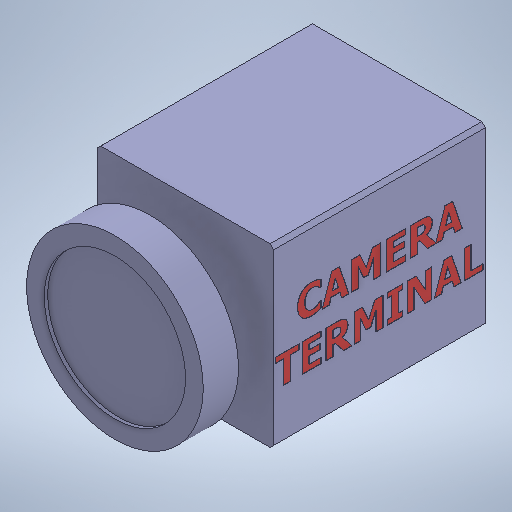
# Autodesk Inventor part: CAMERA
Saved by Autodesk Inventor 2025 (Build 290162000, 162)
## iProperties
Created: 2024-09-26
Part Number: CAMERA
Material: ABS Plastic
Document SubType Name: Modeling
Designer: DMIADX
Density: 1.06 g/cm^3
Appearance: Slate Blue
Author: DMIADX
Autodesk Inventor part; units mm, degrees
ref_plane "YZ Plane" through (0, 0, 0) normal (1, 0, 0) x (0, 1, 0)
ref_plane "XZ Plane" through (0, 0, 0) normal (0, 1, 0) x (-1, 0, 0)
ref_plane "XY Plane" through (0, 0, 0) normal (0, 0, 1) x (1, 0, 0)
sketch "Sketch1" plane through (0, 0, 0) normal (0, 0, 1) x (1, 0, 0)
  line L0 (25, -25) -> (-25, -25)
  line L1 (-25, -25) -> (-25, 25)
  line L2 (-25, 25) -> (25, 25)
  line L3 (25, 25) -> (25, -25)
  line L4 (25, -25) -> (-25, 25) construction
  line L5 (-25, -25) -> (25, 25) construction
  point P0 (0, 0)
  dimension "d0" = 50
  dimension "d1" = 50
  constraints: 12 end point, 2 midpoint, 2 parallel, 1 horizontal, 1 perpendicular
  measures "d0" distance of L0.end L1.end
  measures "d1" distance of L1.end L2.end
extrude "Extrusion1" add sketch "Sketch1" along normal blind 60
chamfer "Chamfer1" distance 1 angle 45 4 edges at (25, 25, 30) (-25, 25, 30) (-25, -25, 30) (25, -25, 30)
sketch "Sketch2" plane through (0, 0, 60) normal (0, 0, 1) x (1, 0, 0)
  circle A0 centre (0, 0) radius 25
  line L0 (24, 25) -> (-24, 25) projected
  circle A1 centre (0, 0) radius 10
  dimension "d7" = 20
  constraints: 2 centre point, 2 coincident, 1 tangent
  measures "d7" diameter of A1
extrude "Extrusion2" add sketch "Sketch2" along normal blind 20 contours A0 | A1
extrude "Extrusion3" cut sketch "Sketch2" along normal blind 10
sketch "Sketch3" plane through (0, 0, 80) normal (0, 0, 1) x (1, 0, 0)
  circle A0 centre (0, 0) radius 20
  constraints: 1 centre point, 1 coincident
extrude "Extrusion4" cut sketch "Sketch3" against normal blind 1
sketch "Sketch4" plane through (25, -24, 0) normal (1, 0, 0) x (0, 0, -1)
  line L0 (-60, 49) -> (0, 49) construction
  line L1 (0, 49) -> (0, -1) construction
  line L2 (0, -1) -> (-60, -1) construction
  line L3 (-60, -1) -> (-60, 49) construction
  line L4 (0, 0) -> (0, 48) projected
  spline S0 degree 2 poles (-49.2512, 26.3525) (-51.0535, 26.3525) (-53.1669, 28.5308) (-53.1669, 30.5016) knots 0 0 0 1 2 2 2
  spline S1 degree 2 poles (-53.1669, 30.5016) (-53.1669, 32.4011) (-51.047, 34.6637) (-49.2447, 34.6637) knots 0 0 0 1 2 2 2
  spline S2 degree 2 poles (-49.2447, 34.6637) (-48.7715, 34.6637) (-48.0065, 34.5535) (-47.6564, 34.4627) knots 0 0 0 1 2 2 2
  spline S3 degree 2 poles (-47.6564, 34.4627) (-47.3841, 34.3784) (-46.7423, 34.0997) (-46.5413, 33.9959) knots 0 0 0 1 2 2 2
  line L5 (-46.5413, 33.9959) -> (-46.5413, 32.0899)
  line L6 (-46.5413, 32.0899) -> (-46.7423, 32.0899)
  spline S4 degree 2 poles (-46.7423, 32.0899) (-46.8914, 32.2196) (-47.3323, 32.5827) (-47.611, 32.7512) knots 0 0 0 1 2 2 2
  spline S5 degree 2 poles (-47.611, 32.7512) (-47.8898, 32.9263) (-48.5575, 33.1661) (-48.9271, 33.1661) knots 0 0 0 1 2 2 2
  spline S6 degree 2 poles (-48.9271, 33.1661) (-49.3614, 33.1661) (-50.081, 32.8938) (-50.4117, 32.5502) knots 0 0 0 1 2 2 2
  spline S7 degree 2 poles (-50.4117, 32.5502) (-50.7099, 32.2455) (-51.0924, 31.2018) (-51.0924, 30.4951) knots 0 0 0 1 2 2 2
  spline S8 degree 2 poles (-51.0924, 30.4951) (-51.0924, 29.7496) (-50.6969, 28.7318) (-50.3728, 28.4206) knots 0 0 0 1 2 2 2
  spline S9 degree 2 poles (-50.3728, 28.4206) (-50.0616, 28.1159) (-49.2966, 27.8501) (-48.9141, 27.8501) knots 0 0 0 1 2 2 2
  spline S10 degree 2 poles (-48.9141, 27.8501) (-48.5186, 27.8501) (-47.799, 28.1159) (-47.5527, 28.278) knots 0 0 0 1 2 2 2
  spline S11 degree 2 poles (-47.5527, 28.278) (-47.2804, 28.44) (-46.872, 28.7836) (-46.7229, 28.9198) knots 0 0 0 1 2 2 2
  line L7 (-46.7229, 28.9198) -> (-46.5413, 28.9198)
  line L8 (-46.5413, 28.9198) -> (-46.5413, 27.0397)
  spline S12 degree 2 poles (-46.5413, 27.0397) (-46.7618, 26.936) (-47.3387, 26.6767) (-47.6499, 26.5859) knots 0 0 0 1 2 2 2
  spline S13 degree 2 poles (-47.6499, 26.5859) (-48.0259, 26.4692) (-48.6807, 26.3525) (-49.2512, 26.3525) knots 0 0 0 1 2 2 2
  line L9 (-46.2172, 26.5081) -> (-43.5138, 34.5081)
  line L10 (-43.5138, 34.5081) -> (-41.3225, 34.5081)
  line L11 (-41.3225, 34.5081) -> (-38.6191, 26.5081)
  line L12 (-38.6191, 26.5081) -> (-40.6872, 26.5081)
  line L13 (-40.6872, 26.5081) -> (-41.1864, 28.1418)
  line L14 (-41.1864, 28.1418) -> (-43.7018, 28.1418)
  line L15 (-43.7018, 28.1418) -> (-44.2075, 26.5081)
  line L16 (-44.2075, 26.5081) -> (-46.2172, 26.5081)
  line L17 (-41.6272, 29.594) -> (-42.4441, 32.2391)
  line L18 (-42.4441, 32.2391) -> (-43.2674, 29.594)
  line L19 (-43.2674, 29.594) -> (-41.6272, 29.594)
  line L20 (-29.6532, 26.5081) -> (-31.6499, 26.5081)
  line L21 (-31.6499, 26.5081) -> (-31.6499, 31.8112)
  line L22 (-31.6499, 31.8112) -> (-33.1021, 28.3882)
  line L23 (-33.1021, 28.3882) -> (-34.4765, 28.3882)
  line L24 (-34.4765, 28.3882) -> (-35.9287, 31.8112)
  line L25 (-35.9287, 31.8112) -> (-35.9287, 26.5081)
  line L26 (-35.9287, 26.5081) -> (-37.8217, 26.5081)
  line L27 (-37.8217, 26.5081) -> (-37.8217, 34.5081)
  line L28 (-37.8217, 34.5081) -> (-35.5073, 34.5081)
  line L29 (-35.5073, 34.5081) -> (-33.731, 30.56)
  line L30 (-33.731, 30.56) -> (-31.9676, 34.5081)
  line L31 (-31.9676, 34.5081) -> (-29.6532, 34.5081)
  line L32 (-29.6532, 34.5081) -> (-29.6532, 26.5081)
  line L33 (-27.9935, 26.5081) -> (-27.9935, 34.5081)
  line L34 (-27.9935, 34.5081) -> (-22.5867, 34.5081)
  line L35 (-22.5867, 34.5081) -> (-22.5867, 32.9846)
  line L36 (-22.5867, 32.9846) -> (-25.9968, 32.9846)
  line L37 (-25.9968, 32.9846) -> (-25.9968, 31.5778)
  line L38 (-25.9968, 31.5778) -> (-22.8525, 31.5778)
  line L39 (-22.8525, 31.5778) -> (-22.8525, 30.0543)
  line L40 (-22.8525, 30.0543) -> (-25.9968, 30.0543)
  line L41 (-25.9968, 30.0543) -> (-25.9968, 28.0316)
  line L42 (-25.9968, 28.0316) -> (-22.5867, 28.0316)
  line L43 (-22.5867, 28.0316) -> (-22.5867, 26.5081)
  line L44 (-22.5867, 26.5081) -> (-27.9935, 26.5081)
  line L45 (-13.8347, 26.5081) -> (-16.2788, 26.5081)
  line L46 (-16.2788, 26.5081) -> (-18.5024, 29.4449)
  line L47 (-18.5024, 29.4449) -> (-19.2285, 29.4449)
  line L48 (-19.2285, 29.4449) -> (-19.2285, 26.5081)
  line L49 (-19.2285, 26.5081) -> (-21.2253, 26.5081)
  line L50 (-21.2253, 26.5081) -> (-21.2253, 34.5081)
  line L51 (-21.2253, 34.5081) -> (-18.0097, 34.5081)
  spline S14 degree 2 poles (-18.0097, 34.5081) (-17.342, 34.5081) (-16.3566, 34.3395) (-15.9352, 34.0802) knots 0 0 0 1 2 2 2
  spline S15 degree 2 poles (-15.9352, 34.0802) (-15.5073, 33.8079) (-15.0016, 32.9587) (-15.0016, 32.3104) knots 0 0 0 1 2 2 2
  spline S16 degree 2 poles (-15.0016, 32.3104) (-15.0016, 31.3963) (-15.8314, 30.2488) (-16.5251, 29.9117) knots 0 0 0 1 2 2 2
  line L52 (-16.5251, 29.9117) -> (-13.8347, 26.5081)
  spline S17 degree 2 poles (-17.0632, 32.0575) (-17.0632, 32.3622) (-17.2966, 32.7966) (-17.5624, 32.9133) knots 0 0 0 1 2 2 2
  spline S18 degree 2 poles (-17.5624, 32.9133) (-17.7504, 32.9911) (-18.2107, 33.0365) (-18.5543, 33.0365) knots 0 0 0 1 2 2 2
  line L53 (-18.5543, 33.0365) -> (-19.2285, 33.0365)
  line L54 (-19.2285, 33.0365) -> (-19.2285, 30.8841)
  line L55 (-19.2285, 30.8841) -> (-18.6515, 30.8841)
  spline S19 degree 2 poles (-18.6515, 30.8841) (-18.2366, 30.8841) (-17.6467, 30.9878) (-17.4457, 31.1499) knots 0 0 0 1 2 2 2
  spline S20 degree 2 poles (-17.4457, 31.1499) (-17.2512, 31.3055) (-17.0632, 31.7204) (-17.0632, 32.0575) knots 0 0 0 1 2 2 2
  line L56 (-14.1005, 26.5081) -> (-11.3971, 34.5081)
  line L57 (-11.3971, 34.5081) -> (-9.2058, 34.5081)
  line L58 (-9.2058, 34.5081) -> (-6.5024, 26.5081)
  line L59 (-6.5024, 26.5081) -> (-8.5705, 26.5081)
  line L60 (-8.5705, 26.5081) -> (-9.0697, 28.1418)
  line L61 (-9.0697, 28.1418) -> (-11.5851, 28.1418)
  line L62 (-11.5851, 28.1418) -> (-12.0908, 26.5081)
  line L63 (-12.0908, 26.5081) -> (-14.1005, 26.5081)
  line L64 (-9.5105, 29.594) -> (-10.3274, 32.2391)
  line L65 (-10.3274, 32.2391) -> (-11.1507, 29.594)
  line L66 (-11.1507, 29.594) -> (-9.5105, 29.594)
  line L67 (-57.1053, 13.3363) -> (-57.1053, 19.8128)
  line L68 (-57.1053, 19.8128) -> (-59.4716, 19.8128)
  line L69 (-59.4716, 19.8128) -> (-59.4716, 21.3363)
  line L70 (-59.4716, 21.3363) -> (-52.7293, 21.3363)
  line L71 (-52.7293, 21.3363) -> (-52.7293, 19.8128)
  line L72 (-52.7293, 19.8128) -> (-55.0956, 19.8128)
  line L73 (-55.0956, 19.8128) -> (-55.0956, 13.3363)
  line L74 (-55.0956, 13.3363) -> (-57.1053, 13.3363)
  line L75 (-51.906, 13.3363) -> (-51.906, 21.3363)
  line L76 (-51.906, 21.3363) -> (-46.4992, 21.3363)
  line L77 (-46.4992, 21.3363) -> (-46.4992, 19.8128)
  line L78 (-46.4992, 19.8128) -> (-49.9092, 19.8128)
  line L79 (-49.9092, 19.8128) -> (-49.9092, 18.406)
  line L80 (-49.9092, 18.406) -> (-46.765, 18.406)
  line L81 (-46.765, 18.406) -> (-46.765, 16.8825)
  line L82 (-46.765, 16.8825) -> (-49.9092, 16.8825)
  line L83 (-49.9092, 16.8825) -> (-49.9092, 14.8598)
  line L84 (-49.9092, 14.8598) -> (-46.4992, 14.8598)
  line L85 (-46.4992, 14.8598) -> (-46.4992, 13.3363)
  line L86 (-46.4992, 13.3363) -> (-51.906, 13.3363)
  line L87 (-37.7472, 13.3363) -> (-40.1912, 13.3363)
  line L88 (-40.1912, 13.3363) -> (-42.4149, 16.2731)
  line L89 (-42.4149, 16.2731) -> (-43.141, 16.2731)
  line L90 (-43.141, 16.2731) -> (-43.141, 13.3363)
  line L91 (-43.141, 13.3363) -> (-45.1378, 13.3363)
  line L92 (-45.1378, 13.3363) -> (-45.1378, 21.3363)
  line L93 (-45.1378, 21.3363) -> (-41.9222, 21.3363)
  spline S21 degree 2 poles (-41.9222, 21.3363) (-41.2545, 21.3363) (-40.269, 21.1678) (-39.8477, 20.9084) knots 0 0 0 1 2 2 2
  spline S22 degree 2 poles (-39.8477, 20.9084) (-39.4198, 20.6361) (-38.9141, 19.7869) (-38.9141, 19.1386) knots 0 0 0 1 2 2 2
  spline S23 degree 2 poles (-38.9141, 19.1386) (-38.9141, 18.2245) (-39.7439, 17.077) (-40.4376, 16.7399) knots 0 0 0 1 2 2 2
  line L94 (-40.4376, 16.7399) -> (-37.7472, 13.3363)
  spline S24 degree 2 poles (-40.9757, 18.8857) (-40.9757, 19.1904) (-41.2091, 19.6248) (-41.4749, 19.7415) knots 0 0 0 1 2 2 2
  spline S25 degree 2 poles (-41.4749, 19.7415) (-41.6629, 19.8193) (-42.1232, 19.8647) (-42.4668, 19.8647) knots 0 0 0 1 2 2 2
  line L95 (-42.4668, 19.8647) -> (-43.141, 19.8647)
  line L96 (-43.141, 19.8647) -> (-43.141, 17.7123)
  line L97 (-43.141, 17.7123) -> (-42.564, 17.7123)
  spline S26 degree 2 poles (-42.564, 17.7123) (-42.1491, 17.7123) (-41.5592, 17.8161) (-41.3582, 17.9781) knots 0 0 0 1 2 2 2
  spline S27 degree 2 poles (-41.3582, 17.9781) (-41.1637, 18.1337) (-40.9757, 18.5486) (-40.9757, 18.8857) knots 0 0 0 1 2 2 2
  line L98 (-28.9822, 13.3363) -> (-30.9789, 13.3363)
  line L99 (-30.9789, 13.3363) -> (-30.9789, 18.6394)
  line L100 (-30.9789, 18.6394) -> (-32.4311, 15.2164)
  line L101 (-32.4311, 15.2164) -> (-33.8055, 15.2164)
  line L102 (-33.8055, 15.2164) -> (-35.2577, 18.6394)
  line L103 (-35.2577, 18.6394) -> (-35.2577, 13.3363)
  line L104 (-35.2577, 13.3363) -> (-37.1507, 13.3363)
  line L105 (-37.1507, 13.3363) -> (-37.1507, 21.3363)
  line L106 (-37.1507, 21.3363) -> (-34.8363, 21.3363)
  line L107 (-34.8363, 21.3363) -> (-33.06, 17.3882)
  line L108 (-33.06, 17.3882) -> (-31.2966, 21.3363)
  line L109 (-31.2966, 21.3363) -> (-28.9822, 21.3363)
  line L110 (-28.9822, 21.3363) -> (-28.9822, 13.3363)
  line L111 (-23.342, 13.3363) -> (-27.6467, 13.3363)
  line L112 (-27.6467, 13.3363) -> (-27.6467, 14.7302)
  line L113 (-27.6467, 14.7302) -> (-26.4992, 14.7302)
  line L114 (-26.4992, 14.7302) -> (-26.4992, 19.9425)
  line L115 (-26.4992, 19.9425) -> (-27.6467, 19.9425)
  line L116 (-27.6467, 19.9425) -> (-27.6467, 21.3363)
  line L117 (-27.6467, 21.3363) -> (-23.342, 21.3363)
  line L118 (-23.342, 21.3363) -> (-23.342, 19.9425)
  line L119 (-23.342, 19.9425) -> (-24.4895, 19.9425)
  line L120 (-24.4895, 19.9425) -> (-24.4895, 14.7302)
  line L121 (-24.4895, 14.7302) -> (-23.342, 14.7302)
  line L122 (-23.342, 14.7302) -> (-23.342, 13.3363)
  line L123 (-15.154, 13.3363) -> (-17.0859, 13.3363)
  line L124 (-17.0859, 13.3363) -> (-20.1718, 18.9117)
  line L125 (-20.1718, 18.9117) -> (-20.1718, 13.3363)
  line L126 (-20.1718, 13.3363) -> (-22.0065, 13.3363)
  line L127 (-22.0065, 13.3363) -> (-22.0065, 21.3363)
  line L128 (-22.0065, 21.3363) -> (-19.543, 21.3363)
  line L129 (-19.543, 21.3363) -> (-16.9887, 16.7528)
  line L130 (-16.9887, 16.7528) -> (-16.9887, 21.3363)
  line L131 (-16.9887, 21.3363) -> (-15.154, 21.3363)
  line L132 (-15.154, 21.3363) -> (-15.154, 13.3363)
  line L133 (-14.389, 13.3363) -> (-11.6856, 21.3363)
  line L134 (-11.6856, 21.3363) -> (-9.4943, 21.3363)
  line L135 (-9.4943, 21.3363) -> (-6.7909, 13.3363)
  line L136 (-6.7909, 13.3363) -> (-8.859, 13.3363)
  line L137 (-8.859, 13.3363) -> (-9.3582, 14.97)
  line L138 (-9.3582, 14.97) -> (-11.8736, 14.97)
  line L139 (-11.8736, 14.97) -> (-12.3793, 13.3363)
  line L140 (-12.3793, 13.3363) -> (-14.389, 13.3363)
  line L141 (-9.799, 16.4222) -> (-10.6159, 19.0673)
  line L142 (-10.6159, 19.0673) -> (-11.4392, 16.4222)
  line L143 (-11.4392, 16.4222) -> (-9.799, 16.4222)
  line L144 (-0.658, 13.3363) -> (-5.9935, 13.3363)
  line L145 (-5.9935, 13.3363) -> (-5.9935, 21.3363)
  line L146 (-5.9935, 21.3363) -> (-3.9838, 21.3363)
  line L147 (-3.9838, 21.3363) -> (-3.9838, 14.8598)
  line L148 (-3.9838, 14.8598) -> (-0.658, 14.8598)
  line L149 (-0.658, 14.8598) -> (-0.658, 13.3363)
  point P0 (0, 24)
  point P1 (0, 24)
  point P2 (0, 24)
  dimension "d14" = 60
  dimension "d15" = 0
  dimension "d16" = 50
  dimension "d17" = 25
  constraints: 2 midpoint, 2 other
  measures "d14" distance of L1.end L2.end
  measures "d15" horizontal distance of point (0, 24) L1.end
  measures "d16" distance between parallel lines of L2 L0
  measures "d17" distance from line of point (0, 24) L0
emboss "Emboss1" sketch "Sketch4" operation cut depth 0.1 direction (-1, 0, 0)
sketch "Sketch5" plane through (-25, -24, 0) normal (-1, 0, 0) x (0, 0, 1)
  line L0 (0, 49) -> (60, 49) construction
  line L1 (60, 49) -> (60, -1) construction
  line L2 (60, -1) -> (0, -1) construction
  line L3 (0, -1) -> (0, 49) construction
  line L4 (0, -1) -> (60, -1) projected
  line L5 (60, 48) -> (60, 0) projected
  spline S0 degree 2 poles (10.7488, 26.3525) (8.9465, 26.3525) (6.8331, 28.5308) (6.8331, 30.5016) knots 0 0 0 1 2 2 2
  spline S1 degree 2 poles (6.8331, 30.5016) (6.8331, 32.4011) (8.953, 34.6637) (10.7553, 34.6637) knots 0 0 0 1 2 2 2
  spline S2 degree 2 poles (10.7553, 34.6637) (11.2285, 34.6637) (11.9935, 34.5535) (12.3436, 34.4627) knots 0 0 0 1 2 2 2
  spline S3 degree 2 poles (12.3436, 34.4627) (12.6159, 34.3784) (13.2577, 34.0997) (13.4587, 33.9959) knots 0 0 0 1 2 2 2
  line L6 (13.4587, 33.9959) -> (13.4587, 32.0899)
  line L7 (13.4587, 32.0899) -> (13.2577, 32.0899)
  spline S4 degree 2 poles (13.2577, 32.0899) (13.1086, 32.2196) (12.6677, 32.5827) (12.389, 32.7512) knots 0 0 0 1 2 2 2
  spline S5 degree 2 poles (12.389, 32.7512) (12.1102, 32.9263) (11.4425, 33.1661) (11.0729, 33.1661) knots 0 0 0 1 2 2 2
  spline S6 degree 2 poles (11.0729, 33.1661) (10.6386, 33.1661) (9.919, 32.8938) (9.5883, 32.5502) knots 0 0 0 1 2 2 2
  spline S7 degree 2 poles (9.5883, 32.5502) (9.2901, 32.2455) (8.9076, 31.2018) (8.9076, 30.4951) knots 0 0 0 1 2 2 2
  spline S8 degree 2 poles (8.9076, 30.4951) (8.9076, 29.7496) (9.3031, 28.7318) (9.6272, 28.4206) knots 0 0 0 1 2 2 2
  spline S9 degree 2 poles (9.6272, 28.4206) (9.9384, 28.1159) (10.7034, 27.8501) (11.0859, 27.8501) knots 0 0 0 1 2 2 2
  spline S10 degree 2 poles (11.0859, 27.8501) (11.4814, 27.8501) (12.201, 28.1159) (12.4473, 28.278) knots 0 0 0 1 2 2 2
  spline S11 degree 2 poles (12.4473, 28.278) (12.7196, 28.44) (13.128, 28.7836) (13.2771, 28.9198) knots 0 0 0 1 2 2 2
  line L8 (13.2771, 28.9198) -> (13.4587, 28.9198)
  line L9 (13.4587, 28.9198) -> (13.4587, 27.0397)
  spline S12 degree 2 poles (13.4587, 27.0397) (13.2382, 26.936) (12.6613, 26.6767) (12.3501, 26.5859) knots 0 0 0 1 2 2 2
  spline S13 degree 2 poles (12.3501, 26.5859) (11.9741, 26.4692) (11.3193, 26.3525) (10.7488, 26.3525) knots 0 0 0 1 2 2 2
  line L10 (13.7828, 26.5081) -> (16.4862, 34.5081)
  line L11 (16.4862, 34.5081) -> (18.6775, 34.5081)
  line L12 (18.6775, 34.5081) -> (21.3809, 26.5081)
  line L13 (21.3809, 26.5081) -> (19.3128, 26.5081)
  line L14 (19.3128, 26.5081) -> (18.8136, 28.1418)
  line L15 (18.8136, 28.1418) -> (16.2982, 28.1418)
  line L16 (16.2982, 28.1418) -> (15.7925, 26.5081)
  line L17 (15.7925, 26.5081) -> (13.7828, 26.5081)
  line L18 (18.3728, 29.594) -> (17.5559, 32.2391)
  line L19 (17.5559, 32.2391) -> (16.7326, 29.594)
  line L20 (16.7326, 29.594) -> (18.3728, 29.594)
  line L21 (30.3468, 26.5081) -> (28.3501, 26.5081)
  line L22 (28.3501, 26.5081) -> (28.3501, 31.8112)
  line L23 (28.3501, 31.8112) -> (26.8979, 28.3882)
  line L24 (26.8979, 28.3882) -> (25.5235, 28.3882)
  line L25 (25.5235, 28.3882) -> (24.0713, 31.8112)
  line L26 (24.0713, 31.8112) -> (24.0713, 26.5081)
  line L27 (24.0713, 26.5081) -> (22.1783, 26.5081)
  line L28 (22.1783, 26.5081) -> (22.1783, 34.5081)
  line L29 (22.1783, 34.5081) -> (24.4927, 34.5081)
  line L30 (24.4927, 34.5081) -> (26.269, 30.56)
  line L31 (26.269, 30.56) -> (28.0324, 34.5081)
  line L32 (28.0324, 34.5081) -> (30.3468, 34.5081)
  line L33 (30.3468, 34.5081) -> (30.3468, 26.5081)
  line L34 (32.0065, 26.5081) -> (32.0065, 34.5081)
  line L35 (32.0065, 34.5081) -> (37.4133, 34.5081)
  line L36 (37.4133, 34.5081) -> (37.4133, 32.9846)
  line L37 (37.4133, 32.9846) -> (34.0032, 32.9846)
  line L38 (34.0032, 32.9846) -> (34.0032, 31.5778)
  line L39 (34.0032, 31.5778) -> (37.1475, 31.5778)
  line L40 (37.1475, 31.5778) -> (37.1475, 30.0543)
  line L41 (37.1475, 30.0543) -> (34.0032, 30.0543)
  line L42 (34.0032, 30.0543) -> (34.0032, 28.0316)
  line L43 (34.0032, 28.0316) -> (37.4133, 28.0316)
  line L44 (37.4133, 28.0316) -> (37.4133, 26.5081)
  line L45 (37.4133, 26.5081) -> (32.0065, 26.5081)
  line L46 (46.1653, 26.5081) -> (43.7212, 26.5081)
  line L47 (43.7212, 26.5081) -> (41.4976, 29.4449)
  line L48 (41.4976, 29.4449) -> (40.7715, 29.4449)
  line L49 (40.7715, 29.4449) -> (40.7715, 26.5081)
  line L50 (40.7715, 26.5081) -> (38.7747, 26.5081)
  line L51 (38.7747, 26.5081) -> (38.7747, 34.5081)
  line L52 (38.7747, 34.5081) -> (41.9903, 34.5081)
  spline S14 degree 2 poles (41.9903, 34.5081) (42.658, 34.5081) (43.6434, 34.3395) (44.0648, 34.0802) knots 0 0 0 1 2 2 2
  spline S15 degree 2 poles (44.0648, 34.0802) (44.4927, 33.8079) (44.9984, 32.9587) (44.9984, 32.3104) knots 0 0 0 1 2 2 2
  spline S16 degree 2 poles (44.9984, 32.3104) (44.9984, 31.3963) (44.1686, 30.2488) (43.4749, 29.9117) knots 0 0 0 1 2 2 2
  line L53 (43.4749, 29.9117) -> (46.1653, 26.5081)
  spline S17 degree 2 poles (42.9368, 32.0575) (42.9368, 32.3622) (42.7034, 32.7966) (42.4376, 32.9133) knots 0 0 0 1 2 2 2
  spline S18 degree 2 poles (42.4376, 32.9133) (42.2496, 32.9911) (41.7893, 33.0365) (41.4457, 33.0365) knots 0 0 0 1 2 2 2
  line L54 (41.4457, 33.0365) -> (40.7715, 33.0365)
  line L55 (40.7715, 33.0365) -> (40.7715, 30.8841)
  line L56 (40.7715, 30.8841) -> (41.3485, 30.8841)
  spline S19 degree 2 poles (41.3485, 30.8841) (41.7634, 30.8841) (42.3533, 30.9878) (42.5543, 31.1499) knots 0 0 0 1 2 2 2
  spline S20 degree 2 poles (42.5543, 31.1499) (42.7488, 31.3055) (42.9368, 31.7204) (42.9368, 32.0575) knots 0 0 0 1 2 2 2
  line L57 (45.8995, 26.5081) -> (48.6029, 34.5081)
  line L58 (48.6029, 34.5081) -> (50.7942, 34.5081)
  line L59 (50.7942, 34.5081) -> (53.4976, 26.5081)
  line L60 (53.4976, 26.5081) -> (51.4295, 26.5081)
  line L61 (51.4295, 26.5081) -> (50.9303, 28.1418)
  line L62 (50.9303, 28.1418) -> (48.4149, 28.1418)
  line L63 (48.4149, 28.1418) -> (47.9092, 26.5081)
  line L64 (47.9092, 26.5081) -> (45.8995, 26.5081)
  line L65 (50.4895, 29.594) -> (49.6726, 32.2391)
  line L66 (49.6726, 32.2391) -> (48.8493, 29.594)
  line L67 (48.8493, 29.594) -> (50.4895, 29.594)
  line L68 (2.8947, 13.3363) -> (2.8947, 19.8128)
  line L69 (2.8947, 19.8128) -> (0.5284, 19.8128)
  line L70 (0.5284, 19.8128) -> (0.5284, 21.3363)
  line L71 (0.5284, 21.3363) -> (7.2707, 21.3363)
  line L72 (7.2707, 21.3363) -> (7.2707, 19.8128)
  line L73 (7.2707, 19.8128) -> (4.9044, 19.8128)
  line L74 (4.9044, 19.8128) -> (4.9044, 13.3363)
  line L75 (4.9044, 13.3363) -> (2.8947, 13.3363)
  line L76 (8.094, 13.3363) -> (8.094, 21.3363)
  line L77 (8.094, 21.3363) -> (13.5008, 21.3363)
  line L78 (13.5008, 21.3363) -> (13.5008, 19.8128)
  line L79 (13.5008, 19.8128) -> (10.0908, 19.8128)
  line L80 (10.0908, 19.8128) -> (10.0908, 18.406)
  line L81 (10.0908, 18.406) -> (13.235, 18.406)
  line L82 (13.235, 18.406) -> (13.235, 16.8825)
  line L83 (13.235, 16.8825) -> (10.0908, 16.8825)
  line L84 (10.0908, 16.8825) -> (10.0908, 14.8598)
  line L85 (10.0908, 14.8598) -> (13.5008, 14.8598)
  line L86 (13.5008, 14.8598) -> (13.5008, 13.3363)
  line L87 (13.5008, 13.3363) -> (8.094, 13.3363)
  line L88 (22.2528, 13.3363) -> (19.8088, 13.3363)
  line L89 (19.8088, 13.3363) -> (17.5851, 16.2731)
  line L90 (17.5851, 16.2731) -> (16.859, 16.2731)
  line L91 (16.859, 16.2731) -> (16.859, 13.3363)
  line L92 (16.859, 13.3363) -> (14.8622, 13.3363)
  line L93 (14.8622, 13.3363) -> (14.8622, 21.3363)
  line L94 (14.8622, 21.3363) -> (18.0778, 21.3363)
  spline S21 degree 2 poles (18.0778, 21.3363) (18.7455, 21.3363) (19.731, 21.1678) (20.1523, 20.9084) knots 0 0 0 1 2 2 2
  spline S22 degree 2 poles (20.1523, 20.9084) (20.5802, 20.6361) (21.0859, 19.7869) (21.0859, 19.1386) knots 0 0 0 1 2 2 2
  spline S23 degree 2 poles (21.0859, 19.1386) (21.0859, 18.2245) (20.2561, 17.077) (19.5624, 16.7399) knots 0 0 0 1 2 2 2
  line L95 (19.5624, 16.7399) -> (22.2528, 13.3363)
  spline S24 degree 2 poles (19.0243, 18.8857) (19.0243, 19.1904) (18.7909, 19.6248) (18.5251, 19.7415) knots 0 0 0 1 2 2 2
  spline S25 degree 2 poles (18.5251, 19.7415) (18.3371, 19.8193) (17.8768, 19.8647) (17.5332, 19.8647) knots 0 0 0 1 2 2 2
  line L96 (17.5332, 19.8647) -> (16.859, 19.8647)
  line L97 (16.859, 19.8647) -> (16.859, 17.7123)
  line L98 (16.859, 17.7123) -> (17.436, 17.7123)
  spline S26 degree 2 poles (17.436, 17.7123) (17.8509, 17.7123) (18.4408, 17.8161) (18.6418, 17.9781) knots 0 0 0 1 2 2 2
  spline S27 degree 2 poles (18.6418, 17.9781) (18.8363, 18.1337) (19.0243, 18.5486) (19.0243, 18.8857) knots 0 0 0 1 2 2 2
  line L99 (31.0178, 13.3363) -> (29.0211, 13.3363)
  line L100 (29.0211, 13.3363) -> (29.0211, 18.6394)
  line L101 (29.0211, 18.6394) -> (27.5689, 15.2164)
  line L102 (27.5689, 15.2164) -> (26.1945, 15.2164)
  line L103 (26.1945, 15.2164) -> (24.7423, 18.6394)
  line L104 (24.7423, 18.6394) -> (24.7423, 13.3363)
  line L105 (24.7423, 13.3363) -> (22.8493, 13.3363)
  line L106 (22.8493, 13.3363) -> (22.8493, 21.3363)
  line L107 (22.8493, 21.3363) -> (25.1637, 21.3363)
  line L108 (25.1637, 21.3363) -> (26.94, 17.3882)
  line L109 (26.94, 17.3882) -> (28.7034, 21.3363)
  line L110 (28.7034, 21.3363) -> (31.0178, 21.3363)
  line L111 (31.0178, 21.3363) -> (31.0178, 13.3363)
  line L112 (36.658, 13.3363) -> (32.3533, 13.3363)
  line L113 (32.3533, 13.3363) -> (32.3533, 14.7302)
  line L114 (32.3533, 14.7302) -> (33.5008, 14.7302)
  line L115 (33.5008, 14.7302) -> (33.5008, 19.9425)
  line L116 (33.5008, 19.9425) -> (32.3533, 19.9425)
  line L117 (32.3533, 19.9425) -> (32.3533, 21.3363)
  line L118 (32.3533, 21.3363) -> (36.658, 21.3363)
  line L119 (36.658, 21.3363) -> (36.658, 19.9425)
  line L120 (36.658, 19.9425) -> (35.5105, 19.9425)
  line L121 (35.5105, 19.9425) -> (35.5105, 14.7302)
  line L122 (35.5105, 14.7302) -> (36.658, 14.7302)
  line L123 (36.658, 14.7302) -> (36.658, 13.3363)
  line L124 (44.846, 13.3363) -> (42.9141, 13.3363)
  line L125 (42.9141, 13.3363) -> (39.8282, 18.9117)
  line L126 (39.8282, 18.9117) -> (39.8282, 13.3363)
  line L127 (39.8282, 13.3363) -> (37.9935, 13.3363)
  line L128 (37.9935, 13.3363) -> (37.9935, 21.3363)
  line L129 (37.9935, 21.3363) -> (40.457, 21.3363)
  line L130 (40.457, 21.3363) -> (43.0113, 16.7528)
  line L131 (43.0113, 16.7528) -> (43.0113, 21.3363)
  line L132 (43.0113, 21.3363) -> (44.846, 21.3363)
  line L133 (44.846, 21.3363) -> (44.846, 13.3363)
  line L134 (45.611, 13.3363) -> (48.3144, 21.3363)
  line L135 (48.3144, 21.3363) -> (50.5057, 21.3363)
  line L136 (50.5057, 21.3363) -> (53.2091, 13.3363)
  line L137 (53.2091, 13.3363) -> (51.141, 13.3363)
  line L138 (51.141, 13.3363) -> (50.6418, 14.97)
  line L139 (50.6418, 14.97) -> (48.1264, 14.97)
  line L140 (48.1264, 14.97) -> (47.6207, 13.3363)
  line L141 (47.6207, 13.3363) -> (45.611, 13.3363)
  line L142 (50.201, 16.4222) -> (49.3841, 19.0673)
  line L143 (49.3841, 19.0673) -> (48.5608, 16.4222)
  line L144 (48.5608, 16.4222) -> (50.201, 16.4222)
  line L145 (59.342, 13.3363) -> (54.0065, 13.3363)
  line L146 (54.0065, 13.3363) -> (54.0065, 21.3363)
  line L147 (54.0065, 21.3363) -> (56.0162, 21.3363)
  line L148 (56.0162, 21.3363) -> (56.0162, 14.8598)
  line L149 (56.0162, 14.8598) -> (59.342, 14.8598)
  line L150 (59.342, 14.8598) -> (59.342, 13.3363)
  point P0 (0, 24)
  point P1 (19.3189, -2.8778)
  point P2 (60, 24)
  point P3 (53.9887, 24)
  dimension "d20" = 60
  dimension "d21" = 0
  dimension "d22" = 50
  dimension "d23" = 25
  dimension "d24" = 0
  dimension "d25" = 0
  constraints: 2 other
  measures "d20" distance of L1.end L2.end
  measures "d21" horizontal distance of point (60, 24) L1.end
  measures "d22" distance between parallel lines of L2 L0
  measures "d23" distance from line of point (53.989, 24) L0
  measures "d24" distance between parallel lines of L4 L2
  measures "d25" distance between parallel lines of L5 L1
emboss "Emboss2" sketch "Sketch5" operation cut depth 0.1 direction (1, 0, 0)
sketch "Sketch6" plane through (0, 0, 0) normal (0, 0, -1) x (-1, 0, 0)
  line L0 (-20, 20) -> (20, 20) construction
  line L1 (20, 20) -> (20, -20) construction
  line L2 (20, -20) -> (-20, -20) construction
  line L3 (-20, -20) -> (-20, 20) construction
  spline S0 degree 2 poles (-14.6791, 1.7938) (-16.0533, 1.7938) (-17.6648, 3.4547) (-17.6648, 4.9575) knots 0 0 0 1 2 2 2
  spline S1 degree 2 poles (-17.6648, 4.9575) (-17.6648, 6.4059) (-16.0483, 8.1311) (-14.6741, 8.1311) knots 0 0 0 1 2 2 2
  spline S2 degree 2 poles (-14.6741, 8.1311) (-14.3133, 8.1311) (-13.7299, 8.047) (-13.463, 7.9778) knots 0 0 0 1 2 2 2
  spline S3 degree 2 poles (-13.463, 7.9778) (-13.2554, 7.9136) (-12.766, 7.701) (-12.6128, 7.6219) knots 0 0 0 1 2 2 2
  line L4 (-12.6128, 7.6219) -> (-12.6128, 6.1686)
  line L5 (-12.6128, 6.1686) -> (-12.766, 6.1686)
  spline S4 degree 2 poles (-12.766, 6.1686) (-12.8797, 6.2675) (-13.2158, 6.5443) (-13.4284, 6.6728) knots 0 0 0 1 2 2 2
  spline S5 degree 2 poles (-13.4284, 6.6728) (-13.641, 6.8063) (-14.1501, 6.9892) (-14.4319, 6.9892) knots 0 0 0 1 2 2 2
  spline S6 degree 2 poles (-14.4319, 6.9892) (-14.7631, 6.9892) (-15.3118, 6.7816) (-15.5639, 6.5196) knots 0 0 0 1 2 2 2
  spline S7 degree 2 poles (-15.5639, 6.5196) (-15.7913, 6.2872) (-16.0829, 5.4914) (-16.0829, 4.9525) knots 0 0 0 1 2 2 2
  spline S8 degree 2 poles (-16.0829, 4.9525) (-16.0829, 4.3841) (-15.7814, 3.608) (-15.5342, 3.3707) knots 0 0 0 1 2 2 2
  spline S9 degree 2 poles (-15.5342, 3.3707) (-15.297, 3.1384) (-14.7137, 2.9357) (-14.422, 2.9357) knots 0 0 0 1 2 2 2
  spline S10 degree 2 poles (-14.422, 2.9357) (-14.1205, 2.9357) (-13.5718, 3.1384) (-13.3839, 3.2619) knots 0 0 0 1 2 2 2
  spline S11 degree 2 poles (-13.3839, 3.2619) (-13.1763, 3.3855) (-12.8649, 3.6475) (-12.7512, 3.7513) knots 0 0 0 1 2 2 2
  line L6 (-12.7512, 3.7513) -> (-12.6128, 3.7513)
  line L7 (-12.6128, 3.7513) -> (-12.6128, 2.3178)
  spline S12 degree 2 poles (-12.6128, 2.3178) (-12.7808, 2.2387) (-13.2208, 2.041) (-13.4581, 1.9717) knots 0 0 0 1 2 2 2
  spline S13 degree 2 poles (-13.4581, 1.9717) (-13.7448, 1.8828) (-14.244, 1.7938) (-14.6791, 1.7938) knots 0 0 0 1 2 2 2
  line L8 (-12.3656, 1.9124) -> (-10.3043, 8.0124)
  line L9 (-10.3043, 8.0124) -> (-8.6334, 8.0124)
  line L10 (-8.6334, 8.0124) -> (-6.5721, 1.9124)
  line L11 (-6.5721, 1.9124) -> (-8.149, 1.9124)
  line L12 (-8.149, 1.9124) -> (-8.5296, 3.1581)
  line L13 (-8.5296, 3.1581) -> (-10.4476, 3.1581)
  line L14 (-10.4476, 3.1581) -> (-10.8332, 1.9124)
  line L15 (-10.8332, 1.9124) -> (-12.3656, 1.9124)
  line L16 (-8.8658, 4.2654) -> (-9.4886, 6.2823)
  line L17 (-9.4886, 6.2823) -> (-10.1164, 4.2654)
  line L18 (-10.1164, 4.2654) -> (-8.8658, 4.2654)
  line L19 (0.2645, 1.9124) -> (-1.2581, 1.9124)
  line L20 (-1.2581, 1.9124) -> (-1.2581, 5.956)
  line L21 (-1.2581, 5.956) -> (-2.3654, 3.346)
  line L22 (-2.3654, 3.346) -> (-3.4133, 3.346)
  line L23 (-3.4133, 3.346) -> (-4.5206, 5.956)
  line L24 (-4.5206, 5.956) -> (-4.5206, 1.9124)
  line L25 (-4.5206, 1.9124) -> (-5.9641, 1.9124)
  line L26 (-5.9641, 1.9124) -> (-5.9641, 8.0124)
  line L27 (-5.9641, 8.0124) -> (-4.1993, 8.0124)
  line L28 (-4.1993, 8.0124) -> (-2.8449, 5.002)
  line L29 (-2.8449, 5.002) -> (-1.5003, 8.0124)
  line L30 (-1.5003, 8.0124) -> (0.2645, 8.0124)
  line L31 (0.2645, 8.0124) -> (0.2645, 1.9124)
  line L32 (1.5299, 1.9124) -> (1.5299, 8.0124)
  line L33 (1.5299, 8.0124) -> (5.6526, 8.0124)
  line L34 (5.6526, 8.0124) -> (5.6526, 6.8508)
  line L35 (5.6526, 6.8508) -> (3.0525, 6.8508)
  line L36 (3.0525, 6.8508) -> (3.0525, 5.7781)
  line L37 (3.0525, 5.7781) -> (5.45, 5.7781)
  line L38 (5.45, 5.7781) -> (5.45, 4.6164)
  line L39 (5.45, 4.6164) -> (3.0525, 4.6164)
  line L40 (3.0525, 4.6164) -> (3.0525, 3.0741)
  line L41 (3.0525, 3.0741) -> (5.6526, 3.0741)
  line L42 (5.6526, 3.0741) -> (5.6526, 1.9124)
  line L43 (5.6526, 1.9124) -> (1.5299, 1.9124)
  line L44 (12.3261, 1.9124) -> (10.4624, 1.9124)
  line L45 (10.4624, 1.9124) -> (8.7669, 4.1517)
  line L46 (8.7669, 4.1517) -> (8.2132, 4.1517)
  line L47 (8.2132, 4.1517) -> (8.2132, 1.9124)
  line L48 (8.2132, 1.9124) -> (6.6907, 1.9124)
  line L49 (6.6907, 1.9124) -> (6.6907, 8.0124)
  line L50 (6.6907, 8.0124) -> (9.1426, 8.0124)
  spline S14 degree 2 poles (9.1426, 8.0124) (9.6517, 8.0124) (10.4031, 7.8839) (10.7244, 7.6862) knots 0 0 0 1 2 2 2
  spline S15 degree 2 poles (10.7244, 7.6862) (11.0507, 7.4786) (11.4363, 6.831) (11.4363, 6.3367) knots 0 0 0 1 2 2 2
  spline S16 degree 2 poles (11.4363, 6.3367) (11.4363, 5.6397) (10.8035, 4.7647) (10.2746, 4.5076) knots 0 0 0 1 2 2 2
  line L51 (10.2746, 4.5076) -> (12.3261, 1.9124)
  spline S17 degree 2 poles (9.8643, 6.1439) (9.8643, 6.3762) (9.6863, 6.7074) (9.4837, 6.7964) knots 0 0 0 1 2 2 2
  spline S18 degree 2 poles (9.4837, 6.7964) (9.3403, 6.8557) (8.9893, 6.8903) (8.7274, 6.8903) knots 0 0 0 1 2 2 2
  line L52 (8.7274, 6.8903) -> (8.2132, 6.8903)
  line L53 (8.2132, 6.8903) -> (8.2132, 5.2491)
  line L54 (8.2132, 5.2491) -> (8.6532, 5.2491)
  spline S19 degree 2 poles (8.6532, 5.2491) (8.9696, 5.2491) (9.4194, 5.3282) (9.5727, 5.4518) knots 0 0 0 1 2 2 2
  spline S20 degree 2 poles (9.5727, 5.4518) (9.7209, 5.5704) (9.8643, 5.8868) (9.8643, 6.1439) knots 0 0 0 1 2 2 2
  line L55 (12.1234, 1.9124) -> (14.1847, 8.0124)
  line L56 (14.1847, 8.0124) -> (15.8556, 8.0124)
  line L57 (15.8556, 8.0124) -> (17.9169, 1.9124)
  line L58 (17.9169, 1.9124) -> (16.34, 1.9124)
  line L59 (16.34, 1.9124) -> (15.9594, 3.1581)
  line L60 (15.9594, 3.1581) -> (14.0414, 3.1581)
  line L61 (14.0414, 3.1581) -> (13.6558, 1.9124)
  line L62 (13.6558, 1.9124) -> (12.1234, 1.9124)
  line L63 (15.6232, 4.2654) -> (15.0004, 6.2823)
  line L64 (15.0004, 6.2823) -> (14.3726, 4.2654)
  line L65 (14.3726, 4.2654) -> (15.6232, 4.2654)
  line L66 (-20.6678, -8.1311) -> (-20.6678, -3.1927)
  line L67 (-20.6678, -3.1927) -> (-22.4721, -3.1927)
  line L68 (-22.4721, -3.1927) -> (-22.4721, -2.0311)
  line L69 (-22.4721, -2.0311) -> (-17.3311, -2.0311)
  line L70 (-17.3311, -2.0311) -> (-17.3311, -3.1927)
  line L71 (-17.3311, -3.1927) -> (-19.1354, -3.1927)
  line L72 (-19.1354, -3.1927) -> (-19.1354, -8.1311)
  line L73 (-19.1354, -8.1311) -> (-20.6678, -8.1311)
  line L74 (-16.7033, -8.1311) -> (-16.7033, -2.0311)
  line L75 (-16.7033, -2.0311) -> (-12.5806, -2.0311)
  line L76 (-12.5806, -2.0311) -> (-12.5806, -3.1927)
  line L77 (-12.5806, -3.1927) -> (-15.1808, -3.1927)
  line L78 (-15.1808, -3.1927) -> (-15.1808, -4.2654)
  line L79 (-15.1808, -4.2654) -> (-12.7833, -4.2654)
  line L80 (-12.7833, -4.2654) -> (-12.7833, -5.4271)
  line L81 (-12.7833, -5.4271) -> (-15.1808, -5.4271)
  line L82 (-15.1808, -5.4271) -> (-15.1808, -6.9694)
  line L83 (-15.1808, -6.9694) -> (-12.5806, -6.9694)
  line L84 (-12.5806, -6.9694) -> (-12.5806, -8.1311)
  line L85 (-12.5806, -8.1311) -> (-16.7033, -8.1311)
  line L86 (-5.9072, -8.1311) -> (-7.7708, -8.1311)
  line L87 (-7.7708, -8.1311) -> (-9.4664, -5.8918)
  line L88 (-9.4664, -5.8918) -> (-10.02, -5.8918)
  line L89 (-10.02, -5.8918) -> (-10.02, -8.1311)
  line L90 (-10.02, -8.1311) -> (-11.5425, -8.1311)
  line L91 (-11.5425, -8.1311) -> (-11.5425, -2.0311)
  line L92 (-11.5425, -2.0311) -> (-9.0907, -2.0311)
  spline S21 degree 2 poles (-9.0907, -2.0311) (-8.5815, -2.0311) (-7.8301, -2.1596) (-7.5088, -2.3573) knots 0 0 0 1 2 2 2
  spline S22 degree 2 poles (-7.5088, -2.3573) (-7.1826, -2.5649) (-6.797, -3.2125) (-6.797, -3.7068) knots 0 0 0 1 2 2 2
  spline S23 degree 2 poles (-6.797, -3.7068) (-6.797, -4.4038) (-7.4297, -5.2788) (-7.9587, -5.5358) knots 0 0 0 1 2 2 2
  line L93 (-7.9587, -5.5358) -> (-5.9072, -8.1311)
  spline S24 degree 2 poles (-8.369, -3.8996) (-8.369, -3.6673) (-8.5469, -3.3361) (-8.7496, -3.2471) knots 0 0 0 1 2 2 2
  spline S25 degree 2 poles (-8.7496, -3.2471) (-8.893, -3.1878) (-9.2439, -3.1532) (-9.5059, -3.1532) knots 0 0 0 1 2 2 2
  line L94 (-9.5059, -3.1532) -> (-10.02, -3.1532)
  line L95 (-10.02, -3.1532) -> (-10.02, -4.7944)
  line L96 (-10.02, -4.7944) -> (-9.5801, -4.7944)
  spline S26 degree 2 poles (-9.5801, -4.7944) (-9.2637, -4.7944) (-8.8139, -4.7153) (-8.6606, -4.5917) knots 0 0 0 1 2 2 2
  spline S27 degree 2 poles (-8.6606, -4.5917) (-8.5123, -4.473) (-8.369, -4.1567) (-8.369, -3.8996) knots 0 0 0 1 2 2 2
  line L97 (0.7761, -8.1311) -> (-0.7464, -8.1311)
  line L98 (-0.7464, -8.1311) -> (-0.7464, -4.0875)
  line L99 (-0.7464, -4.0875) -> (-1.8537, -6.6975)
  line L100 (-1.8537, -6.6975) -> (-2.9017, -6.6975)
  line L101 (-2.9017, -6.6975) -> (-4.009, -4.0875)
  line L102 (-4.009, -4.0875) -> (-4.009, -8.1311)
  line L103 (-4.009, -8.1311) -> (-5.4524, -8.1311)
  line L104 (-5.4524, -8.1311) -> (-5.4524, -2.0311)
  line L105 (-5.4524, -2.0311) -> (-3.6877, -2.0311)
  line L106 (-3.6877, -2.0311) -> (-2.3332, -5.0415)
  line L107 (-2.3332, -5.0415) -> (-0.9887, -2.0311)
  line L108 (-0.9887, -2.0311) -> (0.7761, -2.0311)
  line L109 (0.7761, -2.0311) -> (0.7761, -8.1311)
  line L110 (5.0767, -8.1311) -> (1.7944, -8.1311)
  line L111 (1.7944, -8.1311) -> (1.7944, -7.0683)
  line L112 (1.7944, -7.0683) -> (2.6694, -7.0683)
  line L113 (2.6694, -7.0683) -> (2.6694, -3.0939)
  line L114 (2.6694, -3.0939) -> (1.7944, -3.0939)
  line L115 (1.7944, -3.0939) -> (1.7944, -2.0311)
  line L116 (1.7944, -2.0311) -> (5.0767, -2.0311)
  line L117 (5.0767, -2.0311) -> (5.0767, -3.0939)
  line L118 (5.0767, -3.0939) -> (4.2018, -3.0939)
  line L119 (4.2018, -3.0939) -> (4.2018, -7.0683)
  line L120 (4.2018, -7.0683) -> (5.0767, -7.0683)
  line L121 (5.0767, -7.0683) -> (5.0767, -8.1311)
  line L122 (11.3201, -8.1311) -> (9.847, -8.1311)
  line L123 (9.847, -8.1311) -> (7.494, -3.8798)
  line L124 (7.494, -3.8798) -> (7.494, -8.1311)
  line L125 (7.494, -8.1311) -> (6.0951, -8.1311)
  line L126 (6.0951, -8.1311) -> (6.0951, -2.0311)
  line L127 (6.0951, -2.0311) -> (7.9735, -2.0311)
  line L128 (7.9735, -2.0311) -> (9.9212, -5.526)
  line L129 (9.9212, -5.526) -> (9.9212, -2.0311)
  line L130 (9.9212, -2.0311) -> (11.3201, -2.0311)
  line L131 (11.3201, -2.0311) -> (11.3201, -8.1311)
  line L132 (11.9034, -8.1311) -> (13.9647, -2.0311)
  line L133 (13.9647, -2.0311) -> (15.6356, -2.0311)
  line L134 (15.6356, -2.0311) -> (17.6969, -8.1311)
  line L135 (17.6969, -8.1311) -> (16.12, -8.1311)
  line L136 (16.12, -8.1311) -> (15.7394, -6.8854)
  line L137 (15.7394, -6.8854) -> (13.8214, -6.8854)
  line L138 (13.8214, -6.8854) -> (13.4358, -8.1311)
  line L139 (13.4358, -8.1311) -> (11.9034, -8.1311)
  line L140 (15.4032, -5.7781) -> (14.7804, -3.7612)
  line L141 (14.7804, -3.7612) -> (14.1526, -5.7781)
  line L142 (14.1526, -5.7781) -> (15.4032, -5.7781)
  line L143 (22.3733, -8.1311) -> (18.3049, -8.1311)
  line L144 (18.3049, -8.1311) -> (18.3049, -2.0311)
  line L145 (18.3049, -2.0311) -> (19.8374, -2.0311)
  line L146 (19.8374, -2.0311) -> (19.8374, -6.9694)
  line L147 (19.8374, -6.9694) -> (22.3733, -6.9694)
  line L148 (22.3733, -6.9694) -> (22.3733, -8.1311)
  point P0 (0, 0)
  dimension "d28" = 40
  dimension "d29" = 20
  dimension "d30" = 40
  dimension "d31" = 20
  constraints: 2 other
  measures "d28" distance between parallel lines of L1 L3
  measures "d29" distance from line of point (0, 0) L3
  measures "d30" distance between parallel lines of L0 L2
  measures "d31" horizontal distance of point (0, 0) L1.end
emboss "Emboss3" sketch "Sketch6" operation cut depth 1 direction (0, 0, 1)
sketch "Sketch7" plane through (0, 0, 0) normal (0, 0, -1) x (-1, 0, 0)
  circle A0 centre (0, 0) radius 23.7272
  line L0 (-24, -25) -> (-25, -24) projected
  line L1 (24, -25) -> (-24, -25) projected
  line L2 (25, -24) -> (24, -25) projected
  line L3 (25, 24) -> (25, -24) projected
  line L4 (24, 25) -> (25, 24) projected
  line L5 (-24, 25) -> (24, 25) projected
  line L6 (-25, 24) -> (-24, 25) projected
  line L7 (-25, -24) -> (-25, 24) projected
  line L8 (8.7669, 4.1517) -> (8.2132, 4.1517) projected
  line L9 (8.2132, 4.1517) -> (8.2132, 1.9124) projected
  line L10 (8.2132, 1.9124) -> (6.6907, 1.9124) projected
  line L11 (6.6907, 1.9124) -> (6.6907, 8.0124) projected
  line L12 (6.6907, 8.0124) -> (9.1426, 8.0124) projected
  line L13 (10.2746, 4.5076) -> (12.1841, 2.092) projected
  line L14 (12.1841, 2.092) -> (14.1847, 8.0124) projected
  line L15 (14.1847, 8.0124) -> (15.8556, 8.0124) projected
  line L16 (15.8556, 8.0124) -> (17.9169, 1.9124) projected
  line L17 (17.9169, 1.9124) -> (16.34, 1.9124) projected
  line L18 (16.34, 1.9124) -> (15.9594, 3.1581) projected
  line L19 (15.9594, 3.1581) -> (14.0414, 3.1581) projected
  line L20 (14.0414, 3.1581) -> (13.6558, 1.9124) projected
  line L21 (13.6558, 1.9124) -> (10.4624, 1.9124) projected
  line L22 (10.4624, 1.9124) -> (8.7669, 4.1517) projected
  line L23 (-12.7512, 3.7513) -> (-12.6128, 3.7513) projected
  line L24 (-12.6128, 3.7513) -> (-12.6128, 2.3178) projected
  line L25 (-12.6128, 7.6219) -> (-12.6128, 6.1686) projected
  line L26 (-12.6128, 6.1686) -> (-12.766, 6.1686) projected
  line L27 (-5.9641, 1.9124) -> (-5.9641, 8.0124) projected
  line L28 (-5.9641, 8.0124) -> (-4.1993, 8.0124) projected
  line L29 (-4.1993, 8.0124) -> (-2.8449, 5.002) projected
  line L30 (-2.8449, 5.002) -> (-1.5003, 8.0124) projected
  line L31 (-1.5003, 8.0124) -> (0.2645, 8.0124) projected
  line L32 (0.2645, 8.0124) -> (0.2645, 1.9124) projected
  line L33 (0.2645, 1.9124) -> (-1.2581, 1.9124) projected
  line L34 (-1.2581, 1.9124) -> (-1.2581, 5.956) projected
  line L35 (-1.2581, 5.956) -> (-2.3654, 3.346) projected
  line L36 (-2.3654, 3.346) -> (-3.4133, 3.346) projected
  line L37 (-3.4133, 3.346) -> (-4.5206, 5.956) projected
  line L38 (-4.5206, 5.956) -> (-4.5206, 1.9124) projected
  line L39 (-4.5206, 1.9124) -> (-5.9641, 1.9124) projected
  line L40 (-10.4476, 3.1581) -> (-10.8332, 1.9124) projected
  line L41 (-10.8332, 1.9124) -> (-12.3656, 1.9124) projected
  line L42 (-12.3656, 1.9124) -> (-10.3043, 8.0124) projected
  line L43 (-10.3043, 8.0124) -> (-8.6334, 8.0124) projected
  line L44 (-8.6334, 8.0124) -> (-6.5721, 1.9124) projected
  line L45 (-6.5721, 1.9124) -> (-8.149, 1.9124) projected
  line L46 (-8.149, 1.9124) -> (-8.5296, 3.1581) projected
  line L47 (-8.5296, 3.1581) -> (-10.4476, 3.1581) projected
  line L48 (3.0525, 4.6164) -> (3.0525, 3.0741) projected
  line L49 (3.0525, 3.0741) -> (5.6526, 3.0741) projected
  line L50 (5.6526, 3.0741) -> (5.6526, 1.9124) projected
  line L51 (5.6526, 1.9124) -> (1.5299, 1.9124) projected
  line L52 (1.5299, 1.9124) -> (1.5299, 8.0124) projected
  line L53 (1.5299, 8.0124) -> (5.6526, 8.0124) projected
  line L54 (5.6526, 8.0124) -> (5.6526, 6.8508) projected
  line L55 (5.6526, 6.8508) -> (3.0525, 6.8508) projected
  line L56 (3.0525, 6.8508) -> (3.0525, 5.7781) projected
  line L57 (3.0525, 5.7781) -> (5.45, 5.7781) projected
  line L58 (5.45, 5.7781) -> (5.45, 4.6164) projected
  line L59 (5.45, 4.6164) -> (3.0525, 4.6164) projected
  constraints: 1 centre point, 1 coincident, 17 other
equation "\"d17\" = 0.5 * d16"
equation "\"d23\" = 0.5 * d22"
equation "\"d29\" = 0.5 * d28"
body "Solid1"
